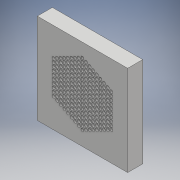
# Autodesk Inventor part: NodeInletVent
Saved by Autodesk Inventor 2017 (Build 210142000, 142)
## iProperties
Created: 2017-10-03
Part Number: NodeInletVent
Material: Generic
Document SubType Name: Modeling
Designer: Kathryn Rosie
Density: 1 g/cm^3
Appearance: Default
Author: Kathryn Rosie
Autodesk Inventor part; units mm, degrees
ref_plane "YZ Plane" through (0, 0, 0) normal (1, 0, 0) x (0, 1, 0)
ref_plane "XZ Plane" through (0, 0, 0) normal (0, 1, 0) x (-1, 0, 0)
ref_plane "XY Plane" through (0, 0, 0) normal (0, 0, 1) x (1, 0, 0)
sketch "Sketch1" plane through (0, 0, 0) normal (0, 1, 0) x (-1, 0, 0)
  line L0 (-75, 75) -> (75, 75)
  line L1 (75, 75) -> (75, -75)
  line L2 (75, -75) -> (-75, -75)
  line L3 (-75, -75) -> (-75, 75)
  line L4 (-75, 75) -> (75, -75) construction
  line L5 (75, 75) -> (-75, -75) construction
  circle A0 centre (0, 52.5) radius 2.5
  line L6 (0, -75) -> (0, 75) construction
  circle A1 centre (0, 46.4) radius 2.5
  circle A2 centre (0, 40.3) radius 2.5
  circle A3 centre (0, 34.2) radius 2.5
  circle A4 centre (0, 28.1) radius 2.5
  circle A5 centre (0, 22) radius 2.5
  circle A6 centre (0, 15.9) radius 2.5
  circle A7 centre (0, 9.8) radius 2.5
  circle A8 centre (0, 3.7) radius 2.5
  circle A9 centre (0, -2.4) radius 2.5
  circle A10 centre (0, -8.5) radius 2.5
  circle A11 centre (0, -14.6) radius 2.5
  circle A12 centre (0, -20.7) radius 2.5
  circle A13 centre (0, -26.8) radius 2.5
  circle A14 centre (0, -32.9) radius 2.5
  circle A15 centre (0, -39) radius 2.5
  circle A16 centre (0, -45.1) radius 2.5
  circle A17 centre (0, -51.2) radius 2.5
  line L7 (-75, 0) -> (75, 0) construction
  circle A18 centre (6, -5.4) radius 2.5
  circle A19 centre (6, -11.5) radius 2.5
  circle A20 centre (6, -17.6) radius 2.5
  circle A21 centre (6, -23.7) radius 2.5
  circle A22 centre (6, -29.8) radius 2.5
  circle A23 centre (6, -35.9) radius 2.5
  circle A24 centre (6, -42) radius 2.5
  circle A25 centre (6, -48.1) radius 2.5
  circle A26 centre (6, 37.3) radius 2.5
  circle A27 centre (6, 31.2) radius 2.5
  circle A28 centre (6, 25.1) radius 2.5
  circle A29 centre (6, 19) radius 2.5
  circle A30 centre (6, 6.8) radius 2.5
  circle A31 centre (6, 0.7) radius 2.5
  circle A32 centre (6, 12.9) radius 2.5
  circle A33 centre (6, 43.4) radius 2.5
  circle A34 centre (6, 49.5) radius 2.5
  circle A35 centre (18, -35.9) radius 2.5
  circle A36 centre (18, -29.8) radius 2.5
  circle A37 centre (18, -42) radius 2.5
  circle A38 centre (18, -23.7) radius 2.5
  circle A39 centre (18, -17.6) radius 2.5
  circle A40 centre (18, -11.5) radius 2.5
  circle A41 centre (18, -5.4) radius 2.5
  circle A42 centre (18, 0.7) radius 2.5
  circle A43 centre (18, 19) radius 2.5
  circle A44 centre (18, 12.9) radius 2.5
  circle A45 centre (18, 6.8) radius 2.5
  circle A46 centre (18, 37.3) radius 2.5
  circle A47 centre (18, 31.2) radius 2.5
  circle A48 centre (18, 25.1) radius 2.5
  circle A49 centre (18, 43.4) radius 2.5
  circle A50 centre (30, -35.9) radius 2.5
  circle A51 centre (30, -29.8) radius 2.5
  circle A52 centre (30, -23.7) radius 2.5
  circle A53 centre (30, -17.6) radius 2.5
  circle A54 centre (30, -11.5) radius 2.5
  circle A55 centre (30, -5.4) radius 2.5
  circle A56 centre (30, 0.7) radius 2.5
  circle A57 centre (30, 19) radius 2.5
  circle A58 centre (30, 12.9) radius 2.5
  circle A59 centre (30, 6.8) radius 2.5
  circle A60 centre (30, 37.3) radius 2.5
  circle A61 centre (30, 31.2) radius 2.5
  circle A62 centre (30, 25.1) radius 2.5
  circle A63 centre (42, -29.8) radius 2.5
  circle A64 centre (42, -23.7) radius 2.5
  circle A65 centre (42, -17.6) radius 2.5
  circle A66 centre (42, -11.5) radius 2.5
  circle A67 centre (42, -5.4) radius 2.5
  circle A68 centre (42, 0.7) radius 2.5
  circle A69 centre (42, 19) radius 2.5
  circle A70 centre (42, 12.9) radius 2.5
  circle A71 centre (42, 6.8) radius 2.5
  circle A72 centre (42, 31.2) radius 2.5
  circle A73 centre (42, 25.1) radius 2.5
  circle A74 centre (-6, -35.9) radius 2.5
  circle A75 centre (-6, -29.8) radius 2.5
  circle A76 centre (-6, -42) radius 2.5
  circle A77 centre (-6, -48.1) radius 2.5
  circle A78 centre (-6, -23.7) radius 2.5
  circle A79 centre (-6, -17.6) radius 2.5
  circle A80 centre (-6, -11.5) radius 2.5
  circle A81 centre (-6, -5.4) radius 2.5
  circle A82 centre (-6, 0.7) radius 2.5
  circle A83 centre (-6, 19) radius 2.5
  circle A84 centre (-6, 12.9) radius 2.5
  circle A85 centre (-6, 6.8) radius 2.5
  circle A86 centre (-6, 37.3) radius 2.5
  circle A87 centre (-6, 31.2) radius 2.5
  circle A88 centre (-6, 25.1) radius 2.5
  circle A89 centre (-6, 43.4) radius 2.5
  circle A90 centre (-6, 49.5) radius 2.5
  circle A91 centre (-18, -35.9) radius 2.5
  circle A92 centre (-18, -29.8) radius 2.5
  circle A93 centre (-18, -42) radius 2.5
  circle A94 centre (-18, -23.7) radius 2.5
  circle A95 centre (-18, -17.6) radius 2.5
  circle A96 centre (-18, -11.5) radius 2.5
  circle A97 centre (-18, -5.4) radius 2.5
  circle A98 centre (-18, 0.7) radius 2.5
  circle A99 centre (-18, 19) radius 2.5
  circle A100 centre (-18, 12.9) radius 2.5
  circle A101 centre (-18, 6.8) radius 2.5
  circle A102 centre (-18, 37.3) radius 2.5
  circle A103 centre (-18, 31.2) radius 2.5
  circle A104 centre (-18, 25.1) radius 2.5
  circle A105 centre (-18, 43.4) radius 2.5
  circle A106 centre (-30, -35.9) radius 2.5
  circle A107 centre (-30, -29.8) radius 2.5
  circle A108 centre (-30, -23.7) radius 2.5
  circle A109 centre (-30, -17.6) radius 2.5
  circle A110 centre (-30, -11.5) radius 2.5
  circle A111 centre (-30, -5.4) radius 2.5
  circle A112 centre (-30, 0.7) radius 2.5
  circle A113 centre (-30, 19) radius 2.5
  circle A114 centre (-30, 12.9) radius 2.5
  circle A115 centre (-30, 6.8) radius 2.5
  circle A116 centre (-30, 37.3) radius 2.5
  circle A117 centre (-30, 31.2) radius 2.5
  circle A118 centre (-30, 25.1) radius 2.5
  circle A119 centre (-42, -29.8) radius 2.5
  circle A120 centre (-42, -23.7) radius 2.5
  circle A121 centre (-42, -17.6) radius 2.5
  circle A122 centre (-42, -11.5) radius 2.5
  circle A123 centre (-42, -5.4) radius 2.5
  circle A124 centre (-42, 0.7) radius 2.5
  circle A125 centre (-42, 19) radius 2.5
  circle A126 centre (-42, 12.9) radius 2.5
  circle A127 centre (-42, 6.8) radius 2.5
  circle A128 centre (-42, 31.2) radius 2.5
  circle A129 centre (-42, 25.1) radius 2.5
  circle A130 centre (-12, 46.4) radius 2.5
  circle A131 centre (-12, 40.3) radius 2.5
  circle A132 centre (-12, 34.2) radius 2.5
  circle A133 centre (-12, 28.1) radius 2.5
  circle A134 centre (-12, 22) radius 2.5
  circle A135 centre (-12, 15.9) radius 2.5
  circle A136 centre (-12, 9.8) radius 2.5
  circle A137 centre (-12, 3.7) radius 2.5
  circle A138 centre (-12, -2.4) radius 2.5
  circle A139 centre (-12, -8.5) radius 2.5
  circle A140 centre (-12, -14.6) radius 2.5
  circle A141 centre (-12, -20.7) radius 2.5
  circle A142 centre (-12, -26.8) radius 2.5
  circle A143 centre (-12, -32.9) radius 2.5
  circle A144 centre (-12, -39) radius 2.5
  circle A145 centre (-12, -45.1) radius 2.5
  circle A146 centre (-24, 40.3) radius 2.5
  circle A147 centre (-24, 34.2) radius 2.5
  circle A148 centre (-24, 28.1) radius 2.5
  circle A149 centre (-24, 22) radius 2.5
  circle A150 centre (-24, 15.9) radius 2.5
  circle A151 centre (-24, 9.8) radius 2.5
  circle A152 centre (-24, 3.7) radius 2.5
  circle A153 centre (-24, -2.4) radius 2.5
  circle A154 centre (-24, -8.5) radius 2.5
  circle A155 centre (-24, -14.6) radius 2.5
  circle A156 centre (-24, -20.7) radius 2.5
  circle A157 centre (-24, -26.8) radius 2.5
  circle A158 centre (-24, -32.9) radius 2.5
  circle A159 centre (-24, -39) radius 2.5
  circle A160 centre (-36, 34.2) radius 2.5
  circle A161 centre (-36, 28.1) radius 2.5
  circle A162 centre (-36, 22) radius 2.5
  circle A163 centre (-36, 15.9) radius 2.5
  circle A164 centre (-36, 9.8) radius 2.5
  circle A165 centre (-36, 3.7) radius 2.5
  circle A166 centre (-36, -2.4) radius 2.5
  circle A167 centre (-36, -8.5) radius 2.5
  circle A168 centre (-36, -14.6) radius 2.5
  circle A169 centre (-36, -20.7) radius 2.5
  circle A170 centre (-36, -26.8) radius 2.5
  circle A171 centre (-36, -32.9) radius 2.5
  circle A172 centre (24, 40.3) radius 2.5
  circle A173 centre (24, 34.2) radius 2.5
  circle A174 centre (24, 28.1) radius 2.5
  circle A175 centre (24, 22) radius 2.5
  circle A176 centre (24, 15.9) radius 2.5
  circle A177 centre (24, 9.8) radius 2.5
  circle A178 centre (24, 3.7) radius 2.5
  circle A179 centre (24, -2.4) radius 2.5
  circle A180 centre (24, -8.5) radius 2.5
  circle A181 centre (24, -14.6) radius 2.5
  circle A182 centre (24, -20.7) radius 2.5
  circle A183 centre (24, -26.8) radius 2.5
  circle A184 centre (24, -32.9) radius 2.5
  circle A185 centre (24, -39) radius 2.5
  circle A186 centre (36, 34.2) radius 2.5
  circle A187 centre (36, 28.1) radius 2.5
  circle A188 centre (36, 22) radius 2.5
  circle A189 centre (36, 15.9) radius 2.5
  circle A190 centre (36, 9.8) radius 2.5
  circle A191 centre (36, 3.7) radius 2.5
  circle A192 centre (36, -2.4) radius 2.5
  circle A193 centre (36, -8.5) radius 2.5
  circle A194 centre (36, -14.6) radius 2.5
  circle A195 centre (36, -20.7) radius 2.5
  circle A196 centre (36, -26.8) radius 2.5
  circle A197 centre (36, -32.9) radius 2.5
  circle A198 centre (48, 15.9) radius 2.5
  circle A199 centre (48, 9.8) radius 2.5
  circle A200 centre (48, 3.7) radius 2.5
  circle A201 centre (48, -2.4) radius 2.5
  circle A202 centre (48, -8.5) radius 2.5
  circle A203 centre (48, -14.6) radius 2.5
  circle A204 centre (48, -20.7) radius 2.5
  circle A205 centre (12, 46.4) radius 2.5
  circle A206 centre (12, 40.3) radius 2.5
  circle A207 centre (12, 34.2) radius 2.5
  circle A208 centre (12, 28.1) radius 2.5
  circle A209 centre (12, 22) radius 2.5
  circle A210 centre (12, 15.9) radius 2.5
  circle A211 centre (12, 9.8) radius 2.5
  circle A212 centre (12, 3.7) radius 2.5
  circle A213 centre (12, -2.4) radius 2.5
  circle A214 centre (12, -8.5) radius 2.5
  circle A215 centre (12, -14.6) radius 2.5
  circle A216 centre (12, -20.7) radius 2.5
  circle A217 centre (12, -26.8) radius 2.5
  circle A218 centre (12, -32.9) radius 2.5
  circle A219 centre (12, -39) radius 2.5
  circle A220 centre (12, -45.1) radius 2.5
  circle A221 centre (-48, 15.9) radius 2.5
  circle A222 centre (-48, 9.8) radius 2.5
  circle A223 centre (-48, 3.7) radius 2.5
  circle A224 centre (-48, -2.4) radius 2.5
  circle A225 centre (-48, -8.5) radius 2.5
  circle A226 centre (-48, -14.6) radius 2.5
  circle A227 centre (-48, -20.7) radius 2.5
  circle A228 centre (48, 21.9) radius 2.5
  circle A229 centre (48, 27.9) radius 2.5
  circle A230 centre (48, -26.7) radius 2.5
  circle A231 centre (-48, 21.9) radius 2.5
  circle A232 centre (-48, 27.9) radius 2.5
  circle A233 centre (-48, -26.7) radius 2.5
  point P0 (0, 0)
  point P1 (6, 49.5)
  point P2 (18, 49.5)
  point P3 (30, 49.5)
  point P4 (42, 49.5)
  point P5 (54, 49.5)
  point P6 (-18, 49.5)
  point P7 (-30, 49.5)
  point P8 (-42, 49.5)
  point P9 (12, 52.5)
  point P10 (24, 52.5)
  point P11 (36, 52.5)
  point P12 (48, 52.5)
  point P13 (-12, 52.5)
  point P14 (-24, 52.5)
  point P15 (-36, 52.5)
  point P16 (-48, 52.5)
  dimension "d1" = 150
  dimension "d2" = 150
  dimension "d3" = 5
  dimension "d6" = 6.1
  dimension "d25" = 6
  dimension "d26" = 3
  dimension "d41" = 12
  dimension "d48" = 12
  dimension "d55" = 12
  dimension "d62" = 12
  dimension "d431" = 6
  dimension "d438" = 6
  dimension "d445" = 6
  dimension "d452" = 6
  constraints: 234 centre point, 16 end point, 5 horizontal, 5 vertical, 4 midpoint, 2 parallel, 1 perpendicular, 1 point on line, 62 other
  measures "d1" distance of L1.end L2.end
  measures "d2" distance of L0.end L1.end
  measures "d3" diameter of A0
  measures "d6" distance of A0.centre A1.centre
  measures "d25" horizontal distance of point (6, 49.5) A0.centre
  measures "d26" vertical distance of point (6, 49.5) A0.centre
  measures "d41" distance of A34.centre point (18, 49.5)
  measures "d48" distance of A34.centre point (-6, 49.5)
  measures "d55" distance of A0.centre point (12, 52.5)
  measures "d62" distance of A0.centre point (-12, 52.5)
  measures "d431" distance of A198.centre A228.centre
  measures "d438" distance of A204.centre A230.centre
  measures "d445" distance of A221.centre A231.centre
  measures "d452" distance of A227.centre A233.centre
extrude "Extrusion2" add sketch "Sketch1" along normal blind 25
body "Solid2"
